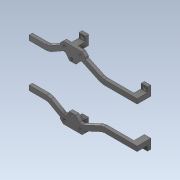
# Autodesk Inventor part: PCB Support
Saved by Autodesk Inventor 2020 (Build 240168000, 168)
## iProperties
Created: 2020-02-29
Part Number: PCB Support
Material: Generic
Document SubType Name: Modeling
Designer: Turing
Density: 1 g/cm^3
Appearance: Smooth - Black
Mass: 40.5652 g
Surface Area: 231.115 cm^2
Volume: 40.5652 cm^3
Author: Turing
Autodesk Inventor part; units mm, degrees
ref_plane "YZ Plane" through (0, 0, 0) normal (1, 0, 0) x (0, 1, 0)
ref_plane "XZ Plane" through (0, 0, 0) normal (0, 1, 0) x (-1, 0, 0)
ref_plane "XY Plane" through (0, 0, 0) normal (0, 0, 1) x (1, 0, 0)
sketch "Sketch1" plane through (0, 0, 0) normal (0, 0, 1) x (1, 0, 0)
  line L0 (-89.294, 31.5003) -> (-89.294, 31.5) projected
  line L1 (-89.294, 31.5) -> (-82.0051, 31.5) projected
  line L2 (-76.3482, 27.5) -> (-82.0051, 31.5) projected
  line L3 (-76.3482, 27.5) -> (-76.3482, -27.5) projected
  line L4 (-82.0051, -31.5) -> (-76.3482, -27.5) projected
  line L5 (-82.0051, -31.5) -> (-89.294, -31.5) projected
  line L6 (-89.294, -31.5) -> (-89.294, -31.5003) projected
  line L7 (-89.294, -31.5003) -> (-94.3529, -43.81) projected
  line L8 (-94.3529, -43.81) -> (-106.8333, -56.2904) projected
  arc A0 (-106.8333, -56.2904) -> (-88.1629, -74.9609) centre (-97.4981, -65.6256) ccw projected
  line L9 (-88.1629, -74.9609) -> (-75.6824, -62.4804) projected
  line L10 (-75.6824, -62.4804) -> (-57.202, -50) projected
  line L11 (-57.202, -50) -> (-38.202, -40) projected
  line L12 (-38.202, -40) -> (-19.202, -50) projected
  line L13 (-19.202, -50) -> (-13.202, -67.65) projected
  line L14 (-13.202, -67.65) -> (-13.202, -85.3001) projected
  arc A1 (-13.202, -85.3001) -> (13.202, -85.3001) centre (0, -85.3001) ccw projected
  line L15 (13.202, -85.3001) -> (13.202, -67.65) projected
  line L16 (13.202, -67.65) -> (19.202, -50) projected
  line L17 (19.202, -50) -> (38.202, -40) projected
  line L18 (38.202, -40) -> (57.202, -50) projected
  line L19 (57.202, -50) -> (75.6824, -62.4804) projected
  line L20 (75.6824, -62.4804) -> (88.1629, -74.9609) projected
  arc A2 (88.1629, -74.9609) -> (106.8333, -56.2904) centre (97.4981, -65.6256) ccw projected
  line L21 (106.8333, -56.2904) -> (94.3529, -43.81) projected
  line L22 (94.3529, -43.81) -> (88.2822, -22.5) projected
  line L23 (88.2822, -22.5) -> (84.2822, -22.5) projected
  line L24 (84.2822, 22.5) -> (84.2822, -22.5) projected
  line L25 (84.2822, 22.5) -> (88.2822, 22.5) projected
  line L26 (88.2822, 22.5) -> (94.3529, 43.81) projected
  line L27 (94.3529, 43.81) -> (106.8333, 56.2904) projected
  arc A3 (106.8333, 56.2904) -> (88.1629, 74.9609) centre (97.4981, 65.6256) ccw projected
  line L28 (88.1629, 74.9609) -> (75.6824, 62.4804) projected
  line L29 (75.6824, 62.4804) -> (57.202, 50) projected
  line L30 (57.202, 50) -> (38.202, 40) projected
  line L31 (38.202, 40) -> (19.202, 50) projected
  line L32 (19.202, 50) -> (13.202, 67.65) projected
  line L33 (13.202, 67.65) -> (13.202, 85.3001) projected
  arc A4 (13.202, 85.3001) -> (-13.202, 85.3001) centre (0, 85.3001) ccw projected
  line L34 (-13.202, 85.3001) -> (-13.202, 67.65) projected
  line L35 (-13.202, 67.65) -> (-19.202, 50) projected
  line L36 (-19.202, 50) -> (-38.202, 40) projected
  line L37 (-38.202, 40) -> (-57.202, 50) projected
  line L38 (-57.202, 50) -> (-75.6824, 62.4804) projected
  line L39 (-75.6824, 62.4804) -> (-88.1629, 74.9609) projected
  arc A5 (-88.1629, 74.9609) -> (-106.8333, 56.2904) centre (-97.4981, 65.6256) ccw projected
  line L40 (-106.8333, 56.2904) -> (-94.3529, 43.81) projected
  line L41 (-94.3529, 43.81) -> (-89.294, 31.5003) projected
  line L42 (103.1549, 64.9185) -> (106.5137, 68.2773) projected
  line L43 (103.1549, 64.9185) -> (104.357, 63.7165) projected
  line L44 (104.357, 63.7165) -> (100.1144, 59.4738) projected
  line L45 (100.1144, 59.4738) -> (83.8509, 43.2104) projected
  line L46 (83.8509, 43.2104) -> (80.3154, 39.6748) projected
  line L47 (80.3154, 39.6748) -> (71.5473, 48.443) projected
  line L48 (71.5473, 48.443) -> (75.0828, 51.9785) projected
  line L49 (75.0828, 51.9785) -> (91.3463, 68.2419) projected
  line L50 (91.3463, 68.2419) -> (95.5889, 72.4846) projected
  line L51 (95.5889, 72.4846) -> (96.791, 71.2825) projected
  line L52 (100.1497, 74.6413) -> (96.791, 71.2825) projected
  line L53 (106.5137, 68.2773) -> (100.1497, 74.6413) projected
  line L54 (4.5, 88.8001) -> (4.5, 93.5501) projected
  line L55 (4.5, 88.8001) -> (6.2, 88.8001) projected
  line L56 (6.2, 88.8001) -> (6.2, 82.8001) projected
  line L57 (6.2, 82.8001) -> (6.2, 59.8001) projected
  line L58 (6.2, 59.8001) -> (6.2, 54.8001) projected
  line L59 (6.2, 54.8001) -> (-6.2, 54.8001) projected
  line L60 (-6.2, 54.8001) -> (-6.2, 59.8001) projected
  line L61 (-6.2, 59.8001) -> (-6.2, 82.8001) projected
  line L62 (-6.2, 82.8001) -> (-6.2, 88.8001) projected
  line L63 (-6.2, 88.8001) -> (-4.5, 88.8001) projected
  line L64 (-4.5, 93.5501) -> (-4.5, 88.8001) projected
  line L65 (4.5, 93.5501) -> (-4.5, 93.5501) projected
  line L66 (-103.1549, -64.9185) -> (-106.5137, -68.2773) projected
  line L67 (-103.1549, -64.9185) -> (-104.357, -63.7165) projected
  line L68 (-104.357, -63.7165) -> (-100.1144, -59.4738) projected
  line L69 (-100.1144, -59.4738) -> (-83.8509, -43.2104) projected
  line L70 (-83.8509, -43.2104) -> (-80.3154, -39.6748) projected
  line L71 (-80.3154, -39.6748) -> (-71.5473, -48.443) projected
  line L72 (-71.5473, -48.443) -> (-75.0828, -51.9785) projected
  line L73 (-75.0828, -51.9785) -> (-91.3463, -68.2419) projected
  line L74 (-91.3463, -68.2419) -> (-95.5889, -72.4846) projected
  line L75 (-95.5889, -72.4846) -> (-96.791, -71.2825) projected
  line L76 (-100.1497, -74.6413) -> (-96.791, -71.2825) projected
  line L77 (-106.5137, -68.2773) -> (-100.1497, -74.6413) projected
  line L78 (-96.791, 71.2825) -> (-100.1497, 74.6413) projected
  line L79 (-96.791, 71.2825) -> (-95.5889, 72.4846) projected
  line L80 (-95.5889, 72.4846) -> (-91.3463, 68.2419) projected
  line L81 (-91.3463, 68.2419) -> (-75.0828, 51.9785) projected
  line L82 (-75.0828, 51.9785) -> (-71.5473, 48.443) projected
  line L83 (-71.5473, 48.443) -> (-80.3154, 39.6748) projected
  line L84 (-80.3154, 39.6748) -> (-83.8509, 43.2104) projected
  line L85 (-83.8509, 43.2104) -> (-100.1144, 59.4738) projected
  line L86 (-100.1144, 59.4738) -> (-104.357, 63.7165) projected
  line L87 (-104.357, 63.7165) -> (-103.1549, 64.9185) projected
  line L88 (-106.5137, 68.2773) -> (-103.1549, 64.9185) projected
  line L89 (-100.1497, 74.6413) -> (-106.5137, 68.2773) projected
  line L90 (-4.5, -88.8001) -> (-4.5, -93.5501) projected
  line L91 (-4.5, -88.8001) -> (-6.2, -88.8001) projected
  line L92 (-6.2, -88.8001) -> (-6.2, -82.8001) projected
  line L93 (-6.2, -82.8001) -> (-6.2, -59.8001) projected
  line L94 (-6.2, -59.8001) -> (-6.2, -54.8001) projected
  line L95 (-6.2, -54.8001) -> (6.2, -54.8001) projected
  line L96 (6.2, -54.8001) -> (6.2, -59.8001) projected
  line L97 (6.2, -59.8001) -> (6.2, -82.8001) projected
  line L98 (6.2, -82.8001) -> (6.2, -88.8001) projected
  line L99 (6.2, -88.8001) -> (4.5, -88.8001) projected
  line L100 (4.5, -93.5501) -> (4.5, -88.8001) projected
  line L101 (-4.5, -93.5501) -> (4.5, -93.5501) projected
  line L102 (96.791, -71.2825) -> (100.1497, -74.6413) projected
  line L103 (96.791, -71.2825) -> (95.5889, -72.4846) projected
  line L104 (95.5889, -72.4846) -> (91.3463, -68.2419) projected
  line L105 (91.3463, -68.2419) -> (75.0828, -51.9785) projected
  line L106 (75.0828, -51.9785) -> (71.5473, -48.443) projected
  line L107 (71.5473, -48.443) -> (80.3154, -39.6748) projected
  line L108 (80.3154, -39.6748) -> (83.8509, -43.2104) projected
  line L109 (83.8509, -43.2104) -> (100.1144, -59.4738) projected
  line L110 (100.1144, -59.4738) -> (104.357, -63.7165) projected
  line L111 (104.357, -63.7165) -> (103.1549, -64.9185) projected
  line L112 (106.5137, -68.2773) -> (103.1549, -64.9185) projected
  line L113 (100.1497, -74.6413) -> (106.5137, -68.2773) projected
  line L114 (60, 22.6) -> (60, 26.6) projected
  line L115 (60, 26.6) -> (-50.9, 26.6) projected
  line L116 (-50.9, 26.6) -> (-50.9, 34.6) projected
  line L117 (-50.9, 34.6) -> (69.1, 34.6) projected
  line L118 (69.1, 34.6) -> (69.1, -34.6) projected
  line L119 (69.1, -34.6) -> (-50.9, -34.6) projected
  line L120 (-50.9, -34.6) -> (-50.9, -26.6) projected
  line L121 (-50.9, -26.6) -> (60, -26.6) projected
  line L122 (60, -26.6) -> (60, -22.6) projected
  line L123 (60, -22.6) -> (-69.1, -22.6) projected
  line L124 (-69.1, -22.6) -> (-69.1, 22.6) projected
  line L125 (-69.1, 22.6) -> (60, 22.6) projected
  line L126 (0, 34.6) -> (0, 54.8001)
  line L127 (-4, 38.7) -> (4, 38.7)
  line L128 (4, 38.7) -> (4, 50.7)
  line L129 (4, 50.7) -> (-4, 50.7)
  line L130 (-4, 50.7) -> (-4, 38.7)
  line L131 (69.1, 0) -> (-69.1, 0)
  line L132 (-4, 44.7) -> (4, 44.7)
  line L133 (73.315, 34.6) -> (81.315, 34.6)
  line L134 (81.315, 34.6) -> (81.315, 22.6)
  line L135 (81.315, 22.6) -> (73.315, 22.6)
  line L136 (73.315, 22.6) -> (73.315, 34.6)
  line L137 (81.315, 28.6) -> (73.315, 28.6)
  line L138 (-4, -38.7) -> (4, -38.7)
  line L139 (4, -38.7) -> (4, -50.7)
  line L140 (4, -50.7) -> (-4, -50.7)
  line L141 (-4, -50.7) -> (-4, -38.7)
  line L142 (-4, -44.7) -> (4, -44.7)
  line L143 (73.315, -34.6) -> (81.315, -34.6)
  line L144 (81.315, -34.6) -> (81.315, -22.6)
  line L145 (81.315, -22.6) -> (73.315, -22.6)
  line L146 (73.315, -22.6) -> (73.315, -34.6)
  line L147 (81.315, -28.6) -> (73.315, -28.6)
  line L148 (81.315, -34.6) -> (73.315, -34.6) projected
  line L149 (73.315, -34.6) -> (73.315, -22.6) projected
  line L150 (73.315, -22.6) -> (81.315, -22.6) projected
  line L151 (81.315, -22.6) -> (81.315, -34.6) projected
  line L152 (4, 38.7) -> (-4, 38.7) projected
  line L153 (-4, 38.7) -> (-4, 50.7) projected
  line L154 (-4, 50.7) -> (4, 50.7) projected
  line L155 (4, 50.7) -> (4, 38.7) projected
  line L156 (4, -50.7) -> (-4, -50.7) projected
  line L157 (-4, -50.7) -> (-4, -38.7) projected
  line L158 (-4, -38.7) -> (4, -38.7) projected
  line L159 (4, -38.7) -> (4, -50.7) projected
  line L160 (81.315, 34.6) -> (81.315, 22.6) projected
  line L161 (81.315, 22.6) -> (73.315, 22.6) projected
  line L162 (73.315, 22.6) -> (73.315, 34.6) projected
  line L163 (73.315, 34.6) -> (81.315, 34.6) projected
  point P0 (0, 0)
  point P1 (0, 44.7)
  point P2 (0, 38.7)
  point P3 (77.315, 34.6)
  dimension "d0" = 8
  dimension "d1" = 20.2001
  dimension "d2" = 12
  dimension "d3" = 8
  dimension "d4" = 12
  dimension "d5" = 4.215
  constraints: 44 end point, 12 symmetric about line, 10 midpoint, 4 parallel, 2 horizontal, 2 horizontal alignment, 2 perpendicular, 1 point on line, 1 vertical alignment
  measures "d0" distance of L127.start L127.end
  measures "d1" distance of L126.start L126.end
  measures "d2" distance of L129.end L127.start
  measures "d3" distance of L134.end L135.end
  measures "d4" distance of L133.end L134.end
  measures "d5" distance between parallel lines of L136 L118
extrude "Extrusion1" add sketch "Sketch1" along normal blind 4 contours L127 L130 L132 L126 | L126 L132 L128 L127 | L132 L130 L129 L126 | L126 L129 L128 L132 | L133 L134 L137 L136 | L137 L134 L135 L136 | L138 L139 L142 L141 | L142 L139 L140 L141 | L146 L147 L144 L143 | L146 L145 L144 L147
sketch "Sketch2" plane through (0, 0, 4) normal (0, 0, 1) x (1, 0, 0)
  line L0 (4, 38.7) -> (4, 50.7) projected
  line L1 (4, 50.7) -> (-4, 50.7) projected
  line L2 (-4, 50.7) -> (-4, 38.7) projected
  line L3 (-4, 38.7) -> (4, 38.7) projected
  line L4 (73.315, 22.6) -> (81.315, 22.6) projected
  line L5 (81.315, 22.6) -> (81.315, 34.6) projected
  line L6 (81.315, 34.6) -> (73.315, 34.6) projected
  line L7 (73.315, 34.6) -> (73.315, 22.6) projected
  line L8 (81.315, -34.6) -> (81.315, -22.6) projected
  line L9 (81.315, -22.6) -> (73.315, -22.6) projected
  line L10 (73.315, -22.6) -> (73.315, -34.6) projected
  line L11 (73.315, -34.6) -> (81.315, -34.6) projected
  line L12 (-4, -50.7) -> (4, -50.7) projected
  line L13 (4, -50.7) -> (4, -38.7) projected
  line L14 (4, -38.7) -> (-4, -38.7) projected
  line L15 (-4, -38.7) -> (-4, -50.7) projected
  line L16 (-4, 38.7) -> (4, 38.7)
  line L17 (4, 38.7) -> (4, 44.7)
  line L18 (4, 44.7) -> (-4, 44.7)
  line L19 (-4, 44.7) -> (-4, 38.7)
  line L20 (-4, -38.7) -> (4, -38.7)
  line L21 (4, -38.7) -> (4, -44.7)
  line L22 (4, -44.7) -> (-4, -44.7)
  line L23 (-4, -44.7) -> (-4, -38.7)
  line L24 (73.315, -22.6) -> (81.315, -22.6)
  line L25 (81.315, -22.6) -> (81.315, -28.6)
  line L26 (81.315, -28.6) -> (73.315, -28.6)
  line L27 (73.315, -28.6) -> (73.315, -22.6)
  line L28 (73.315, 22.6) -> (81.315, 22.6)
  line L29 (81.315, 22.6) -> (81.315, 28.6)
  line L30 (81.315, 28.6) -> (73.315, 28.6)
  line L31 (73.315, 28.6) -> (73.315, 22.6)
  point P0 (0, 0)
  dimension "d8" = 6
  dimension "d9" = 6
  dimension "d10" = 6
  dimension "d11" = 6
  constraints: 32 end point, 10 equal length, 6 perpendicular
  measures "d8" distance of L17.end L0.start
  measures "d9" distance of L30.end L4.start
  measures "d10" distance of L26.end L9.end
  measures "d11" distance of L13.end L21.end
extrude "Extrusion2" add sketch "Sketch2" along normal blind 9 contours L3 L2 L18 L0 | L7 L30 L5 L4 | L26 L10 L9 L8 | L15 L14 L13 L22
sketch "Sketch3" plane through (0, 0, 13) normal (0, 0, 1) x (1, 0, 0)
  line L0 (-4, -44.7) -> (4, -44.7) projected
  line L1 (4, -44.7) -> (4, -38.7) projected
  line L2 (4, -38.7) -> (-4, -38.7) projected
  line L3 (-4, -38.7) -> (-4, -44.7) projected
  line L4 (81.315, -22.6) -> (73.315, -22.6) projected
  line L5 (73.315, -22.6) -> (73.315, -28.6) projected
  line L6 (73.315, -28.6) -> (81.315, -28.6) projected
  line L7 (81.315, -28.6) -> (81.315, -22.6) projected
  line L8 (81.315, 22.6) -> (81.315, 28.6) projected
  line L9 (81.315, 28.6) -> (73.315, 28.6) projected
  line L10 (73.315, 28.6) -> (73.315, 22.6) projected
  line L11 (73.315, 22.6) -> (81.315, 22.6) projected
  line L12 (4, 44.7) -> (-4, 44.7) projected
  line L13 (-4, 44.7) -> (-4, 38.7) projected
  line L14 (-4, 38.7) -> (4, 38.7) projected
  line L15 (4, 38.7) -> (4, 44.7) projected
  line L16 (4, -44.7) -> (38.5266, -28.6)
  line L17 (38.5266, -28.6) -> (73.315, -28.6)
  line L18 (-4, -44.7) -> (4, -44.7)
  line L19 (73.315, -28.6) -> (81.315, -28.6)
  line L20 (81.315, -28.6) -> (81.315, -22.6)
  line L21 (81.315, -22.6) -> (81.315, 28.6)
  line L22 (81.315, 28.6) -> (73.315, 28.6)
  line L23 (73.315, 28.6) -> (38.5266, 28.6)
  line L24 (38.5266, 28.6) -> (4, 44.7)
  line L25 (-4, -44.7) -> (-29.9822, -30)
  line L26 (4, 44.7) -> (-4, 44.7)
  line L27 (-4, 44.7) -> (-29.9822, 30)
  line L28 (-29.9822, -30) -> (-29.9822, 30)
  line L29 (-29.9822, -30) -> (-29.9822, 30)
  line L30 (-29.9822, 30) -> (-59.9822, 30)
  line L31 (-59.9822, 30) -> (-59.9822, -30)
  line L32 (-59.9822, -30) -> (-29.9822, -30)
  point P0 (0, 0)
  dimension "d35" = 81.315
  dimension "d14" = 65
  dimension "d15" = 65
  dimension "d16" = 60.5
  dimension "d17" = 60.5
  dimension "d18" = 119.5
  dimension "d19" = 119.5
  dimension "d20" = 60
  dimension "d21" = 30
  constraints: 34 end point, 6 collinear, 2 parallel, 2 vertical, 1 horizontal, 1 perpendicular, 1 point on line
  measures "d14" angle of L16 L1
  measures "d15" angle of L24 L15
  measures "d16" angle of L3 L25
  measures "d17" angle of L27 L13
  measures "d18" angle of L25 L28
  measures "d19" angle of L28 L27
  measures "d20" distance of L25.end L27.end
  measures "d21" distance of L31.end L25.end
extrude "Extrusion3" add sketch "Sketch3" along normal blind 4
sketch "Sketch4" plane through (0, 0, 4) normal (0, 0, 1) x (1, 0, 0)
  line L0 (4, -44.7) -> (-4, -44.7) projected
  line L1 (-4, -44.7) -> (-4, -50.7) projected
  line L2 (-4, -50.7) -> (4, -50.7) projected
  line L3 (4, -50.7) -> (4, -44.7) projected
  line L4 (81.315, -28.6) -> (73.315, -28.6) projected
  line L5 (73.315, -28.6) -> (73.315, -34.6) projected
  line L6 (73.315, -34.6) -> (81.315, -34.6) projected
  line L7 (81.315, -34.6) -> (81.315, -28.6) projected
  line L8 (-4, 44.7) -> (4, 44.7) projected
  line L9 (4, 44.7) -> (4, 50.7) projected
  line L10 (4, 50.7) -> (-4, 50.7) projected
  line L11 (-4, 50.7) -> (-4, 44.7) projected
  line L12 (73.315, 28.6) -> (81.315, 28.6) projected
  line L13 (81.315, 28.6) -> (81.315, 34.6) projected
  line L14 (81.315, 34.6) -> (73.315, 34.6) projected
  line L15 (73.315, 34.6) -> (73.315, 28.6) projected
  circle A0 centre (0, 47.7) radius 2.8
  circle A1 centre (77.315, 31.6) radius 2.8
  circle A2 centre (77.315, -31.6) radius 2.8
  circle A3 centre (0, -47.7) radius 2.8
  point P0 (0, 0)
  dimension "d24" = 5.6
  dimension "d25" = 5.6
  dimension "d26" = 5.6
  dimension "d27" = 5.6
  dimension "d28" = 3
  dimension "d29" = 4
  dimension "d30" = 66.2
  dimension "d31" = 4
  dimension "d32" = 13.1
  dimension "d33" = 81.315
  dimension "d34" = 82.3
  dimension "d35" = 81.315
  constraints: 4 centre point
  measures "d24" diameter of A0
  measures "d25" diameter of A1
  measures "d26" diameter of A2
  measures "d27" diameter of A3
  measures "d28" distance from line of A1.centre L14
  measures "d29" distance from line of A1.centre L13
  measures "d30" distance from line of A2.centre L14
  measures "d31" distance from line of A2.centre L7
  measures "d32" distance from line of A0.centre L14
  measures "d33" distance from line of A0.centre L7
  measures "d34" distance from line of A3.centre L14
  measures "d35" distance from line of A3.centre L7
extrude "Extrusion4" cut sketch "Sketch4" against normal blind 2.4 contours A0 | A1 | A2 | A3
sketch "Sketch5" plane through (0, 47.7, 1.6) normal (0, 0, 1) x (1, 0, 0)
  circle A0 centre (0, 0) radius 2.8 projected
  circle A1 centre (77.315, -16.1) radius 2.8 projected
  circle A2 centre (77.315, -79.3) radius 2.8 projected
  circle A3 centre (0, -95.4001) radius 2.8 projected
  circle A4 centre (0, 0) radius 1.5
  circle A5 centre (77.315, -16.1) radius 1.5
  circle A6 centre (77.315, -79.3) radius 1.5
  circle A7 centre (0, -95.4001) radius 1.5
  point P0 (0, -47.7)
  dimension "d38" = 3
  dimension "d39" = 3
  dimension "d40" = 3
  dimension "d41" = 3
  constraints: 4 centre point, 4 coincident
  measures "d38" diameter of A4
  measures "d39" diameter of A5
  measures "d40" diameter of A6
  measures "d41" diameter of A7
extrude "Extrusion5" cut sketch "Sketch5" against normal up to surface (1.6 mm away) contours A4 | A5 | A6 | A7
sketch "Sketch6" plane through (0, 0, 17) normal (0, 0, 1) x (1, 0, 0)
  circle A0 centre (0, -47.7) radius 1.5 projected
  line L0 (-4, -50.7) -> (4, -50.7) projected
  line L1 (-4, -38.7) -> (-4, -50.7) projected
  line L2 (4, -38.7) -> (-4, -38.7) projected
  line L3 (4, -50.7) -> (4, -38.7) projected
  circle A1 centre (0, 47.7) radius 1.5 projected
  line L4 (4, 38.7) -> (4, 50.7) projected
  line L5 (-4, 38.7) -> (4, 38.7) projected
  line L6 (-4, 50.7) -> (-4, 38.7) projected
  line L7 (4, 50.7) -> (-4, 50.7) projected
  line L8 (38.5266, 28.6) -> (4, 44.7) projected
  line L9 (4, 44.7) -> (-4, 44.7) projected
  line L10 (-4, 44.7) -> (-29.9822, 30) projected
  line L11 (-29.9822, 30) -> (-59.9822, 30) projected
  line L12 (-59.9822, 30) -> (-59.9822, -30) projected
  line L13 (-59.9822, -30) -> (-29.9822, -30) projected
  line L14 (-29.9822, -30) -> (-4, -44.7) projected
  line L15 (-4, -44.7) -> (4, -44.7) projected
  line L16 (4, -44.7) -> (38.5266, -28.6) projected
  line L17 (38.5266, -28.6) -> (81.315, -28.6) projected
  line L18 (81.315, -28.6) -> (81.315, 28.6) projected
  line L19 (81.315, 28.6) -> (38.5266, 28.6) projected
  point P0 (0, 0)
  point P1 (4, 44.7)
  point P2 (-4, -44.7)
extrude "Extrusion6" add sketch "Sketch6" along normal blind 26 contours L1 L2 L3 L15 | L9 L4 L5 L6
chamfer "Chamfer2" distance 2 angle 45 6 edges at (-59.9822, 30, 15) (-59.9822, -30, 15) (-29.9822, 30, 15) (-29.9822, -30, 15) (38.5266, -28.6, 15) (38.5266, 28.6, 15)
sketch "Sketch13" plane through (0, 0, 43) normal (0, 0, 1) x (1, 0, 0)
  line L0 (4, -44.7) -> (4, -38.7) projected
  line L1 (4, -38.7) -> (-4, -38.7) projected
  line L2 (-4, -38.7) -> (-4, -44.7) projected
  line L3 (-4, -44.7) -> (4, -44.7) projected
  line L4 (-57.9822, -30) -> (-59.9822, -28) projected
  line L5 (-57.9822, -30) -> (-31.9822, -30) projected
  line L6 (-28.2415, -30.9848) -> (-31.9822, -30) projected
  line L7 (-28.2415, -30.9848) -> (-4, -44.7) projected
  line L8 (-4, -38.7) -> (4, -38.7) projected
  line L9 (4, -44.7) -> (36.714, -29.4452) projected
  line L10 (40.5266, -28.6) -> (36.714, -29.4452) projected
  line L11 (40.5266, -28.6) -> (81.315, -28.6) projected
  line L12 (81.315, -28.6) -> (81.315, 28.6) projected
  line L13 (81.315, 28.6) -> (40.5266, 28.6) projected
  line L14 (36.714, 29.4452) -> (40.5266, 28.6) projected
  line L15 (36.714, 29.4452) -> (4, 44.7) projected
  line L16 (4, 38.7) -> (-4, 38.7) projected
  line L17 (-4, 44.7) -> (-28.2415, 30.9848) projected
  line L18 (-31.9822, 30) -> (-28.2415, 30.9848) projected
  line L19 (-31.9822, 30) -> (-57.9822, 30) projected
  line L20 (-59.9822, 28) -> (-57.9822, 30) projected
  line L21 (-59.9822, 28) -> (-59.9822, -28) projected
  line L22 (4, 44.7) -> (-4, 44.7) projected
  line L23 (-4, 44.7) -> (-4, 38.7) projected
  line L24 (-4, 38.7) -> (4, 38.7) projected
  line L25 (4, 38.7) -> (4, 44.7) projected
  line L26 (-4, 38.7) -> (-4, -38.7)
  line L27 (40.5266, 28.6) -> (40.5266, -28.6)
  line L28 (40.5266, -28.6) -> (-25.0734, -28.6)
  line L29 (-25.0734, -28.6) -> (-25.0734, 28.6)
  line L30 (-25.0734, 28.6) -> (40.5266, 28.6)
  line L31 (4, 38.7) -> (4, 28.6)
  line L32 (4, -38.7) -> (4, -28.6)
  line L33 (-25.0734, 0) -> (40.5266, 0)
  line L34 (-20.2734, -23.8) -> (35.7266, -23.8)
  line L35 (-20.2734, -23.8) -> (-20.2734, 23.8)
  circle A0 centre (-20.2734, -23.8) radius 1.25
  circle A1 centre (-20.2734, 23.8) radius 1.25
  line L36 (-20.2734, -23.8) -> (-20.2734, -4.8)
  circle A2 centre (-20.2734, -4.8) radius 1.25
  line L37 (7.7266, -23.8) -> (7.7266, 28.6)
  circle A3 centre (-20.2734, 4.8) radius 1.25
  circle A4 centre (35.7266, -23.8) radius 1.25
  circle A5 centre (35.7266, 23.8) radius 1.25
  circle A6 centre (35.7266, -4.8) radius 1.25
  circle A7 centre (35.7266, 4.8) radius 1.25
  line L38 (-4, -44.7) -> (-4, -38.7) projected
  line L39 (4, -38.7) -> (4, -44.7) projected
  line L40 (4, 44.7) -> (4, 38.7) projected
  line L41 (-4, 38.7) -> (-4, 44.7) projected
  point P0 (0, 0)
  point P1 (-4, 28.6)
  point P2 (-4, -28.6)
  dimension "d105" = 65.6
  dimension "d108" = 56
  dimension "d109" = 47.6
  dimension "d110" = 4.8
  dimension "d111" = 57.2
  dimension "d112" = 4.8
  dimension "d113" = 65.6
  dimension "d114" = 19
  dimension "d115" = 2.5
  dimension "d116" = 2.5
  dimension "d117" = 2.5
  constraints: 24 end point, 8 centre point, 5 symmetric about line, 4 midpoint, 4 perpendicular, 3 coincident, 3 point on line, 2 parallel, 2 vertical, 1 horizontal, 5 other
  measures "d105" distance of L10.start L28.end
  measures "d108" distance of L34.start L34.end
  measures "d109" distance of L34.start L35.end
  measures "d110" distance between parallel lines of L34 L28
  measures "d111" distance of L13.end L10.start
  measures "d112" distance from line of L27 L34.end
  measures "d113" distance of L29.end L13.end
  measures "d114" distance of L36.end L34.start
  measures "d115" diameter of A0
  measures "d116" diameter of A2
  measures "d117" diameter of A1
extrude "Extrusion12" add sketch "Sketch13" against normal blind 4 contours L3 L2 L1 L0 | L1 L26 L28 L32 | L28 L26 L34 L37 L33 L27 | L28 L29 L33 L35 A2 A0 L34 L26 | L33 L37 L30 L27 | L34 A0 L35 A2 L33 L26 | L26 L33 L37 L34 | L33 L26 L30 L37 | L33 L29 L30 L26 | L26 L16 L31 L30 | L25 L16 L23 L22
chamfer "Chamfer3" distance 2 angle 45 12 edges at (4, -28.6, 41) (40.5266, -28.6, 41) (40.5266, 28.6, 41) (4, 28.6, 41) (-4, 28.6, 41) (-25.0734, 28.6, 41) (-25.0734, -28.6, 41) (-4, -28.6, 41) (0, -44.7, 43) (0, 44.7, 43) (0, -38.7, 39) (0, 38.7, 39)
sketch "Sketch14" plane through (-25.0734, -26.6, 43) normal (-1, 0, 0) x (0, 0, 1)
  line L0 (0, 0) -> (-4, 0) projected
  line L1 (0, 53.2) -> (0, 0) projected
  line L2 (-4, 53.2) -> (0, 53.2) projected
  line L3 (-4, 0) -> (-4, 53.2) projected
  line L4 (0, 53.2) -> (0, 0)
  line L5 (0, 26.6) -> (0, 53.2)
  line L6 (0, 39.9) -> (10, 39.9)
  line L7 (0, 29.9) -> (10, 29.9)
  line L8 (10, 29.9) -> (10, 49.9)
  line L9 (10, 49.9) -> (0, 49.9)
  line L10 (0, 49.9) -> (0, 29.9)
  line L11 (0, 29.9) -> (10, 49.9) construction
  line L12 (10, 29.9) -> (0, 49.9) construction
  line L13 (5, 49.9) -> (5, 29.9)
  line L14 (10, 49.9) -> (5, 39.9)
  line L15 (5, 39.9) -> (10, 29.9)
  circle A0 centre (7.5, 44.9) radius 1.25
  circle A1 centre (7.5, 34.9) radius 1.25
  line L16 (0, 49.9) -> (-4, 49.9)
  line L17 (-4, 49.9) -> (-4, 29.9)
  line L18 (-4, 29.9) -> (0, 29.9)
  line L19 (0, 29.9) -> (0, 49.9)
  line L20 (0, 26.6) -> (-4, 26.6)
  line L21 (0, 23.3) -> (10, 23.3)
  line L22 (10, 23.3) -> (10, 3.3)
  line L23 (10, 3.3) -> (0, 3.3)
  circle A2 centre (7.5, 8.3) radius 1.25
  circle A3 centre (7.5, 18.3) radius 1.25
  line L24 (0, 3.3) -> (-4, 3.3)
  line L25 (-4, 3.3) -> (-4, 23.3)
  line L26 (-4, 23.3) -> (0, 23.3)
  point P0 (-43, 26.6)
  point P1 (-4, 23.3)
  point P2 (-4, 3.3)
  point P3 (-4, 49.9)
  point P4 (0, 29.9)
  dimension "d121" = 10
  dimension "d122" = 20
  dimension "d123" = 10
  dimension "d124" = 2.5
  dimension "d125" = 2.5
  dimension "d126" = 20
  constraints: 46 end point, 10 midpoint, 9 symmetric about line, 5 parallel, 4 centre point, 3 collinear, 2 horizontal, 2 perpendicular, 1 point on line, 2 other
  measures "d121" distance of L6.start L6.end
  measures "d122" distance of L8.end L7.end
  measures "d123" distance of L6.start L9.end
  measures "d124" diameter of A0
  measures "d125" diameter of A1
  measures "d126" distance of L17.end L16.end
extrude "Extrusion13" add sketch "Sketch14" along normal blind 4 contours L24 L3 L26 L1 | L1 L21 L22 L23 | L18 L3 L16 L1 | L1 L6 L13 L7 | L1 L9 L13 L6 | L13 L15 A1 L7 | L14 A0 L8 L6 | L13 L9 L14 A0 | L6 L8 L15 A1
chamfer "Chamfer4" distance 2 angle 45 2 edges at (-29.0734, 13.3, 39) (-29.0734, -13.3, 39)
chamfer "Chamfer5" distance 2 angle 45 4 edges at (-25.0734, 23.3, 48) (-25.0734, 3.3, 48) (-25.0734, -3.3, 41) (-25.0734, -23.3, 41)
sketch "Sketch27" plane through (0, 0, 17) normal (0, 0, 1) x (1, 0, 0)
  circle A0 centre (0.0008, 30.4952) radius 1.35 projected
  circle A1 centre (0.0008, -30.3995) radius 1.35 projected
  circle A2 centre (0.0008, 30.4952) radius 1.5
  circle A3 centre (0.0008, -30.3995) radius 1.5
  point P0 (0, 0)
  dimension "d240" = 3
  dimension "d241" = 3
  constraints: 2 centre point, 2 coincident
  measures "d240" diameter of A2
  measures "d241" diameter of A3
extrude "Extrusion26" cut sketch "Sketch27" against normal up to surface (4 mm away) contours A0 | A1 | A2 | A3
sketch "Sketch28" plane through (0, 0, 17) normal (0, 0, 1) x (1, 0, 0)
  line L0 (-57.9822, -30) -> (-59.9822, -28) projected
  line L1 (-57.9822, -30) -> (-31.9822, -30) projected
  line L2 (-28.2415, -30.9848) -> (-31.9822, -30) projected
  line L3 (-28.2415, -30.9848) -> (-4, -44.7) projected
  line L4 (-4, -44.7) -> (-4, -38.7) projected
  line L5 (-4, -38.7) -> (4, -38.7) projected
  line L6 (4, -38.7) -> (4, -44.7) projected
  line L7 (4, -44.7) -> (36.714, -29.4452) projected
  line L8 (40.5266, -28.6) -> (36.714, -29.4452) projected
  line L9 (40.5266, -28.6) -> (81.315, -28.6) projected
  line L10 (81.315, -28.6) -> (81.315, 28.6) projected
  line L11 (81.315, 28.6) -> (40.5266, 28.6) projected
  line L12 (36.714, 29.4452) -> (40.5266, 28.6) projected
  line L13 (36.714, 29.4452) -> (4, 44.7) projected
  line L14 (4, 44.7) -> (4, 38.7) projected
  line L15 (4, 38.7) -> (-4, 38.7) projected
  line L16 (-4, 38.7) -> (-4, 44.7) projected
  line L17 (-4, 44.7) -> (-28.2415, 30.9848) projected
  line L18 (-31.9822, 30) -> (-28.2415, 30.9848) projected
  line L19 (-31.9822, 30) -> (-57.9822, 30) projected
  line L20 (-59.9822, 28) -> (-57.9822, 30) projected
  line L21 (-59.9822, 28) -> (-59.9822, -28) projected
  line L22 (4, -38.7) -> (16.867, -38.7)
  line L23 (16.867, -38.7) -> (16.867, -44.7)
  line L24 (16.867, -44.7) -> (4, -44.7)
  line L25 (-4, -38.7) -> (-14.605, -38.7)
  line L26 (-14.605, -38.7) -> (-14.605, -44.7)
  line L27 (-14.605, -44.7) -> (-4, -44.7)
  line L28 (-59.9822, 0) -> (81.315, 0)
  line L29 (4, 38.7) -> (16.867, 38.7)
  line L30 (16.867, 38.7) -> (16.867, 44.7)
  line L31 (16.867, 44.7) -> (4, 44.7)
  line L32 (-4, 38.7) -> (-14.605, 38.7)
  line L33 (-14.605, 38.7) -> (-14.605, 44.7)
  line L34 (-14.605, 44.7) -> (-4, 44.7)
  point P0 (0, 0)
  constraints: 26 end point, 4 symmetric about line, 3 perpendicular, 2 horizontal, 2 midpoint, 2 point on line, 1 vertical
extrude "Extrusion27" add sketch "Sketch28" against normal up to surface (4 mm away) contours L25 L4 L3 | L3 L27 L26 | L22 L7 L6 | L7 L23 L24 | L33 L34 L17 | L17 L16 L32 | L29 L14 L13 | L13 L31 L30
sketch "Sketch29" plane through (0, 0, 13) normal (0, 0, -1) x (-1, 0, 0)
  line L0 (-36.714, 29.4452) -> (-16.867, 38.7) projected
  line L1 (-40.5266, 28.6) -> (-36.714, 29.4452) projected
  line L2 (-73.315, 28.6) -> (-40.5266, 28.6) projected
  line L3 (-73.315, 28.6) -> (-73.315, 22.6) projected
  line L4 (-73.315, 22.6) -> (-81.315, 22.6) projected
  line L5 (-81.315, -22.6) -> (-81.315, 22.6) projected
  line L6 (-81.315, -22.6) -> (-73.315, -22.6) projected
  line L7 (-73.315, -22.6) -> (-73.315, -28.6) projected
  line L8 (-40.5266, -28.6) -> (-73.315, -28.6) projected
  line L9 (-36.714, -29.4452) -> (-40.5266, -28.6) projected
  line L10 (-16.867, -38.7) -> (-36.714, -29.4452) projected
  line L11 (-16.867, -38.7) -> (-16.867, -44.7) projected
  line L12 (-16.867, -44.7) -> (-4, -44.7) projected
  line L13 (-4, -44.7) -> (-4, -38.7) projected
  line L14 (-4, -38.7) -> (4, -38.7) projected
  line L15 (4, -38.7) -> (4, -44.7) projected
  line L16 (4, -44.7) -> (14.605, -44.7) projected
  line L17 (14.605, -44.7) -> (14.605, -38.7) projected
  line L18 (28.2415, -30.9848) -> (14.605, -38.7) projected
  line L19 (31.9822, -30) -> (28.2415, -30.9848) projected
  line L20 (57.9822, -30) -> (31.9822, -30) projected
  line L21 (59.9822, -28) -> (57.9822, -30) projected
  line L22 (59.9822, 28) -> (59.9822, -28) projected
  line L23 (57.9822, 30) -> (59.9822, 28) projected
  line L24 (31.9822, 30) -> (57.9822, 30) projected
  line L25 (28.2415, 30.9848) -> (31.9822, 30) projected
  line L26 (14.605, 38.7) -> (28.2415, 30.9848) projected
  line L27 (14.605, 38.7) -> (14.605, 44.7) projected
  line L28 (14.605, 44.7) -> (4, 44.7) projected
  line L29 (4, 44.7) -> (4, 38.7) projected
  line L30 (4, 38.7) -> (-4, 38.7) projected
  line L31 (-4, 38.7) -> (-4, 44.7) projected
  line L32 (-4, 44.7) -> (-16.867, 44.7) projected
  line L33 (-16.867, 44.7) -> (-16.867, 38.7) projected
  line L34 (-4, 38.7) -> (-16.867, 38.7)
  line L35 (-10.4335, 38.7) -> (-10.4335, 39.7)
  line L36 (-7.4024, 37.95) -> (-10.4335, 36.2)
  line L37 (-10.4335, 36.2) -> (-13.4646, 37.95)
  line L38 (-13.4646, 37.95) -> (-13.4646, 41.45)
  line L39 (-13.4646, 41.45) -> (-10.4335, 43.2)
  line L40 (-10.4335, 43.2) -> (-7.4024, 41.45)
  line L41 (-7.4024, 41.45) -> (-7.4024, 37.95)
  line L42 (-4, 38.7) -> (-4, 50.7) projected
  line L43 (4, 38.7) -> (14.605, 38.7)
  line L44 (9.3025, 38.7) -> (9.3025, 39.7)
  line L45 (9.3025, 43.2) -> (12.3336, 41.45)
  line L46 (12.3336, 41.45) -> (12.3336, 37.95)
  line L47 (12.3336, 37.95) -> (9.3025, 36.2)
  line L48 (9.3025, 36.2) -> (6.2714, 37.95)
  line L49 (6.2714, 37.95) -> (6.2714, 41.45)
  line L50 (6.2714, 41.45) -> (9.3025, 43.2)
  line L51 (4, 50.7) -> (4, 38.7) projected
  line L52 (59.9822, 0) -> (-81.315, 0)
  line L53 (-7.4024, -37.95) -> (-10.4335, -36.2)
  line L54 (-10.4335, -36.2) -> (-13.4646, -37.95)
  line L55 (-13.4646, -37.95) -> (-13.4646, -41.45)
  line L56 (-13.4646, -41.45) -> (-10.4335, -43.2)
  line L57 (-10.4335, -43.2) -> (-7.4024, -41.45)
  line L58 (-7.4024, -41.45) -> (-7.4024, -37.95)
  line L59 (9.3025, -43.2) -> (12.3336, -41.45)
  line L60 (12.3336, -41.45) -> (12.3336, -37.95)
  line L61 (12.3336, -37.95) -> (9.3025, -36.2)
  line L62 (9.3025, -36.2) -> (6.2714, -37.95)
  line L63 (6.2714, -37.95) -> (6.2714, -41.45)
  line L64 (6.2714, -41.45) -> (9.3025, -43.2)
  point P0 (0, 0)
  dimension "d201" = 1
  dimension "d205" = 7
  dimension "d206" = 1
  dimension "d207" = 7
  constraints: 58 end point, 12 symmetric about line, 4 midpoint, 2 coincident, 2 horizontal, 2 parallel, 2 vertical, 26 other
  measures "d201" distance of L35.start L35.end
  measures "d205" distance of L39.end L36.end
  measures "d206" distance of L44.start L44.end
  measures "d207" distance of L45.start L47.end
extrude "Extrusion28" cut sketch "Sketch29" against normal blind 2.4 contours L38 L39 L40 L41 L34 | L34 L41 L36 L37 L38 | L49 L50 L45 L46 L43 | L43 L46 L47 L48 L49 | L58 L57 L56 L55 L54 L53 | L64 L63 L62 L61 L60 L59
sketch "Sketch30" plane through (0, 0, 13) normal (0, 0, -1) x (-1, 0, 0)
  line L0 (-13.4646, 37.95) -> (-13.4646, 41.45) projected
  line L1 (-10.4335, 36.2) -> (-13.4646, 37.95) projected
  line L2 (-7.4024, 37.95) -> (-10.4335, 36.2) projected
  line L3 (-7.4024, 41.45) -> (-7.4024, 37.95) projected
  line L4 (-10.4335, 43.2) -> (-7.4024, 41.45) projected
  line L5 (-13.4646, 41.45) -> (-10.4335, 43.2) projected
  line L6 (-10.4335, 43.2) -> (-10.4335, 36.2)
  circle A0 centre (-10.4335, 39.7) radius 1.5
  line L7 (6.2714, 37.95) -> (6.2714, 41.45) projected
  line L8 (9.3025, 36.2) -> (6.2714, 37.95) projected
  line L9 (12.3336, 37.95) -> (9.3025, 36.2) projected
  line L10 (12.3336, 41.45) -> (12.3336, 37.95) projected
  line L11 (9.3025, 43.2) -> (12.3336, 41.45) projected
  line L12 (6.2714, 41.45) -> (9.3025, 43.2) projected
  line L13 (9.3025, 43.2) -> (9.3025, 36.2)
  circle A1 centre (9.3025, 39.7) radius 1.5
  line L14 (9.3025, 36.2) -> (6.2714, 37.95) projected
  line L15 (6.2714, 37.95) -> (6.2714, 41.45) projected
  line L16 (6.2714, 41.45) -> (9.3025, 43.2) projected
  line L17 (9.3025, 43.2) -> (12.3336, 41.45) projected
  line L18 (12.3336, 41.45) -> (12.3336, 37.95) projected
  line L19 (12.3336, 37.95) -> (9.3025, 36.2) projected
  line L20 (9.3025, -36.2) -> (12.3336, -37.95) projected
  line L21 (12.3336, -37.95) -> (12.3336, -41.45) projected
  line L22 (12.3336, -41.45) -> (9.3025, -43.2) projected
  line L23 (9.3025, -43.2) -> (6.2714, -41.45) projected
  line L24 (6.2714, -41.45) -> (6.2714, -37.95) projected
  line L25 (6.2714, -37.95) -> (9.3025, -36.2) projected
  line L26 (-10.4335, 36.2) -> (-13.4646, 37.95) projected
  line L27 (-13.4646, 37.95) -> (-13.4646, 41.45) projected
  line L28 (-13.4646, 41.45) -> (-10.4335, 43.2) projected
  line L29 (-10.4335, 43.2) -> (-7.4024, 41.45) projected
  line L30 (-7.4024, 41.45) -> (-7.4024, 37.95) projected
  line L31 (-7.4024, 37.95) -> (-10.4335, 36.2) projected
  line L32 (-10.4335, -43.2) -> (-13.4646, -41.45) projected
  line L33 (-13.4646, -41.45) -> (-13.4646, -37.95) projected
  line L34 (-13.4646, -37.95) -> (-10.4335, -36.2) projected
  line L35 (-10.4335, -36.2) -> (-7.4024, -37.95) projected
  line L36 (-7.4024, -37.95) -> (-7.4024, -41.45) projected
  line L37 (-7.4024, -41.45) -> (-10.4335, -43.2) projected
  line L38 (-36.714, 29.4452) -> (-16.867, 38.7) projected
  line L39 (-40.5266, 28.6) -> (-36.714, 29.4452) projected
  line L40 (-73.315, 28.6) -> (-40.5266, 28.6) projected
  line L41 (-73.315, 28.6) -> (-73.315, 22.6) projected
  line L42 (-73.315, 22.6) -> (-81.315, 22.6) projected
  line L43 (-81.315, -22.6) -> (-81.315, 22.6) projected
  line L44 (-81.315, -22.6) -> (-73.315, -22.6) projected
  line L45 (-73.315, -22.6) -> (-73.315, -28.6) projected
  line L46 (-40.5266, -28.6) -> (-73.315, -28.6) projected
  line L47 (-36.714, -29.4452) -> (-40.5266, -28.6) projected
  line L48 (-16.867, -38.7) -> (-36.714, -29.4452) projected
  line L49 (-16.867, -38.7) -> (-16.867, -44.7) projected
  line L50 (-16.867, -44.7) -> (-4, -44.7) projected
  line L51 (-4, -44.7) -> (-4, -38.7) projected
  line L52 (-4, -38.7) -> (4, -38.7) projected
  line L53 (4, -38.7) -> (4, -44.7) projected
  line L54 (4, -44.7) -> (14.605, -44.7) projected
  line L55 (14.605, -44.7) -> (14.605, -38.7) projected
  line L56 (28.2415, -30.9848) -> (14.605, -38.7) projected
  line L57 (31.9822, -30) -> (28.2415, -30.9848) projected
  line L58 (57.9822, -30) -> (31.9822, -30) projected
  line L59 (59.9822, -28) -> (57.9822, -30) projected
  line L60 (59.9822, 28) -> (59.9822, -28) projected
  line L61 (57.9822, 30) -> (59.9822, 28) projected
  line L62 (31.9822, 30) -> (57.9822, 30) projected
  line L63 (28.2415, 30.9848) -> (31.9822, 30) projected
  line L64 (14.605, 38.7) -> (28.2415, 30.9848) projected
  line L65 (14.605, 38.7) -> (14.605, 44.7) projected
  line L66 (14.605, 44.7) -> (4, 44.7) projected
  line L67 (4, 44.7) -> (4, 38.7) projected
  line L68 (4, 38.7) -> (-4, 38.7) projected
  line L69 (-4, 38.7) -> (-4, 44.7) projected
  line L70 (-4, 44.7) -> (-16.867, 44.7) projected
  line L71 (-16.867, 44.7) -> (-16.867, 38.7) projected
  line L72 (-81.315, 0) -> (59.9822, 0)
  circle A2 centre (-10.4335, -39.7) radius 1.5
  circle A3 centre (9.3025, -39.7) radius 1.5
  point P0 (0, 0)
  dimension "d210" = 3
  dimension "d211" = 3
  constraints: 6 end point, 4 centre point, 4 midpoint, 2 symmetric about line, 2 vertical, 2 other
  measures "d210" diameter of A0
  measures "d211" diameter of A1
extrude "Extrusion29" cut sketch "Sketch30" against normal up to surface (4 mm away) contours A0 L6 | L6 A0 | A1 L13 | L13 A1 | A2 | A3
sketch "Sketch31" plane through (4, 38.7, 17) normal (1, 0, 0) x (0, 0, -1)
  line L0 (0, 6) -> (-24, 6) projected
  line L1 (0, -83.4001) -> (-24, -83.4001) projected
  line L2 (0, 6) -> (0, -83.4001)
  line L3 (0, -83.4001) -> (-45, -83.4001)
  line L4 (-45, -83.4001) -> (-45, 6)
  line L5 (-45, 6) -> (0, 6)
  point P0 (17, -38.7)
  point P1 (-24, -83.4001)
  point P2 (-24, 6)
  dimension "d214" = 45
  constraints: 8 end point, 3 perpendicular, 1 vertical
  measures "d214" distance of L1.start L3.end
extrude "Extrusion30" cut sketch "Sketch31" along normal mid plane 100
chamfer "Chamfer9" distance 4 angle 45 4 edges at (16.867, 44.7, 15) (-14.605, 44.7, 15) (-14.605, -44.7, 15) (16.867, -44.7, 15)
sketch "Sketch32" plane through (0, 0, 17) normal (0, 0, 1) x (1, 0, 0)
  circle A0 centre (-9.3025, 39.7) radius 1.5 projected
  circle A1 centre (10.4335, -39.7) radius 1.5 projected
  circle A2 centre (10.4335, 39.7) radius 1.5 projected
  circle A3 centre (-9.3025, -39.7) radius 1.5 projected
  line L0 (16.867, -40.7) -> (12.867, -44.7) projected
  line L1 (16.867, -40.7) -> (16.867, -38.7) projected
  line L2 (16.867, -38.7) -> (36.714, -29.4452) projected
  line L3 (40.5266, -28.6) -> (36.714, -29.4452) projected
  line L4 (40.5266, -28.6) -> (81.315, -28.6) projected
  line L5 (81.315, -28.6) -> (81.315, 28.6) projected
  line L6 (81.315, 28.6) -> (40.5266, 28.6) projected
  line L7 (36.714, 29.4452) -> (40.5266, 28.6) projected
  line L8 (36.714, 29.4452) -> (16.867, 38.7) projected
  line L9 (16.867, 38.7) -> (16.867, 40.7) projected
  line L10 (12.867, 44.7) -> (16.867, 40.7) projected
  line L11 (12.867, 44.7) -> (-10.605, 44.7) projected
  line L12 (-14.605, 40.7) -> (-10.605, 44.7) projected
  line L13 (-14.605, 40.7) -> (-14.605, 38.7) projected
  line L14 (-14.605, 38.7) -> (-28.2415, 30.9848) projected
  line L15 (-31.9822, 30) -> (-28.2415, 30.9848) projected
  line L16 (-31.9822, 30) -> (-57.9822, 30) projected
  line L17 (-59.9822, 28) -> (-57.9822, 30) projected
  line L18 (-59.9822, 28) -> (-59.9822, -28) projected
  line L19 (-57.9822, -30) -> (-59.9822, -28) projected
  line L20 (-57.9822, -30) -> (-31.9822, -30) projected
  line L21 (-28.2415, -30.9848) -> (-31.9822, -30) projected
  line L22 (-28.2415, -30.9848) -> (-14.605, -38.7) projected
  line L23 (-14.605, -38.7) -> (-14.605, -40.7) projected
  line L24 (-10.605, -44.7) -> (-14.605, -40.7) projected
  line L25 (-10.605, -44.7) -> (12.867, -44.7) projected
  line L26 (81.315, -28.6) -> (81.315, -22.6)
  line L27 (81.315, -22.6) -> (60.315, -22.6)
  line L28 (81.315, 28.6) -> (81.315, 22.6)
  line L29 (81.315, 22.6) -> (60.315, 22.6)
  line L30 (60.315, -22.6) -> (60.315, 22.6)
  line L31 (-31.9822, -30) -> (-52.9822, -30)
  line L32 (-52.9822, -30) -> (-52.9822, 30)
  line L33 (-31.9822, 30) -> (-52.9822, 30)
  line L34 (75.315, -22.6) -> (39.8695, -22.6)
  line L35 (39.8695, -22.6) -> (34.7739, -23.7297)
  line L36 (34.7739, -23.7297) -> (10.867, -34.8776)
  line L37 (10.867, -34.8776) -> (10.867, -38.2148)
  line L38 (10.867, -38.2148) -> (10.3818, -38.7)
  line L39 (10.3818, -38.7) -> (-8.1197, -38.7)
  line L40 (-8.1197, -38.7) -> (-8.605, -38.2148)
  line L41 (-8.605, -38.2148) -> (-8.605, -35.2009)
  line L42 (-8.605, -35.2009) -> (-25.9629, -25.3803)
  line L43 (-25.9629, -25.3803) -> (-31.2056, -24)
  line L44 (-31.2056, -24) -> (-53.9822, -24)
  line L45 (-53.9822, -24) -> (-53.9822, 24)
  line L46 (-53.9822, 24) -> (-31.2056, 24)
  line L47 (-31.2056, 24) -> (-25.9629, 25.3803)
  line L48 (-25.9629, 25.3803) -> (-8.605, 35.2009)
  line L49 (-8.605, 35.2009) -> (-8.605, 38.2148)
  line L50 (-8.605, 38.2148) -> (-8.1197, 38.7)
  line L51 (-8.1197, 38.7) -> (10.3818, 38.7)
  line L52 (10.3818, 38.7) -> (10.867, 38.2148)
  line L53 (10.867, 38.2148) -> (10.867, 34.8776)
  line L54 (10.867, 34.8776) -> (34.7739, 23.7297)
  line L55 (34.7739, 23.7297) -> (39.8695, 22.6)
  line L56 (39.8695, 22.6) -> (75.315, 22.6)
  line L57 (75.315, 22.6) -> (75.315, -22.6)
  line L58 (0.0008, -30.3995) -> (0.0008, -27.3995)
  line L59 (0.0008, -27.3995) -> (5.0008, -27.3995)
  line L60 (5.0008, -27.3995) -> (10.867, -34.8776)
  line L61 (0.0008, -27.3995) -> (-2.9992, -27.3995)
  line L62 (-2.9992, -27.3995) -> (-8.605, -35.2009)
  line L63 (-53.9822, 0) -> (60.315, 0)
  line L64 (0.0008, 27.3995) -> (5.0008, 27.3995)
  line L65 (5.0008, 27.3995) -> (10.867, 34.8776)
  line L66 (0.0008, 27.3995) -> (-2.9992, 27.3995)
  line L67 (-2.9992, 27.3995) -> (-8.605, 35.2009)
  point P0 (0, 0)
  point P1 (-52.9822, 24)
  point P2 (-52.9822, -24)
  dimension "d223" = 6
  dimension "d224" = 21
  dimension "d225" = 6
  dimension "d226" = 21
  dimension "d227" = 21
  dimension "d233" = 6
  dimension "d234" = 3
  dimension "d235" = 5
  dimension "d236" = 3
  constraints: 84 end point, 6 point on line, 3 perpendicular, 3 symmetric about line, 2 midpoint, 1 collinear, 1 horizontal, 1 vertical, 23 other
  measures "d223" distance of L4.end L26.end
  measures "d224" distance of L26.end L27.end
  measures "d225" distance of L5.end L28.end
  measures "d226" distance of L28.end L29.end
  measures "d227" distance of L20.end L31.end
  measures "d233" distance between parallel lines of L4 L34
  measures "d234" distance of L58.start L58.end
  measures "d235" distance of L58.end L59.end
  measures "d236" distance of L58.end L61.end
extrude "Extrusion31" cut sketch "Sketch32" against normal up to surface (4 mm away) contours L60 L59 L61 L62 L42 L43 L44 L32 L63 L30 L34 L35 L36 | L30 L29 L57 L27 | L57 L29 L5 L27 | L63 L32 L46 L47 L48 L67 L66 L64 L65 L54 L55 L56 L30 | L44 L45 L63 L32 | L32 L20 L19 L18 L17 L16 L46 L45 L44 | L63 L45 L46 L32
chamfer "Chamfer11" distance 2 angle 45 4 edges at (10.867, -34.8776, 15) (-8.605, -35.2009, 15) (-8.605, 35.2009, 15) (10.867, 34.8776, 15)
equation "\"d9\" = d8"
equation "\"d10\" = d8"
equation "\"d11\" = d8"
equation "\"d15\" = d14"
equation "\"d17\" = d16"
equation "\"d25\" = d24"
equation "\"d26\" = d24"
equation "\"d27\" = d24"
equation "\"d39\" = d38"
equation "\"d40\" = d38"
equation "\"d41\" = d38"
body "Solid1"
